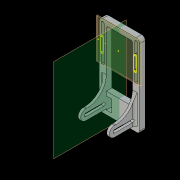
# Autodesk Inventor part: VSlider
Saved by Autodesk Inventor 2022 (Build 260153000, 153)
## iProperties
Created: 2021-12-03
Part Number: VSlider
Material: Generic
Document SubType Name: Modeling
Designer: alber
Density: 1 g/cm^3
Appearance: Default
Mass: 67.3416 g
Surface Area: 306.613 cm^2
Volume: 67.3416 cm^3
Author: alber
Autodesk Inventor part; units mm, degrees
ref_plane "YZ Plane" through (0, 0, 0) normal (1, 0, 0) x (0, 1, 0)
ref_plane "XZ Plane" through (0, 0, 0) normal (0, 1, 0) x (-1, 0, 0)
ref_plane "XY Plane" through (0, 0, 0) normal (0, 0, 1) x (1, 0, 0)
ref_plane "Work Plane1" through (0, 0, 0) normal (0, 0, 1) x (1, 0, 0)
sketch "Sketch1" plane through (0, 0, 0) normal (0, 0, 1) x (1, 0, 0)
  arc A0 (29.8457, -17.7) -> (34.8457, -17.7) centre (32.3457, -17.7) ccw projected
  line L0 (34.8457, 8.3) -> (34.8457, -17.7) projected
  line L1 (29.8457, -17.7) -> (29.8457, 8.3) projected
  arc A1 (34.8457, 8.3) -> (29.8457, 8.3) centre (32.3457, 8.3) ccw projected
  arc A2 (-34.8457, -17.7) -> (-29.8457, -17.7) centre (-32.3457, -17.7) ccw projected
  line L2 (-29.8457, 8.3) -> (-29.8457, -17.7) projected
  line L3 (-34.8457, -17.7) -> (-34.8457, 8.3) projected
  arc A3 (-29.8457, 8.3) -> (-34.8457, 8.3) centre (-32.3457, 8.3) ccw projected
  point P0 (0, 0)
ref_plane "Work Plane2" through (0, 0, -2) normal (0, 0, -1) x (-1, 0, 0)
sketch "Sketch2" plane through (0, 0, -2) normal (0, 0, -1) x (-1, 0, 0)
  arc A0 (-24.3457, -33) -> (-22.3457, -35) centre (-22.3457, -33) ccw projected
  line L0 (-24.3457, -33) -> (-24.3457, -31.7) projected
  arc A1 (-24.3457, -31.7) -> (-31.3457, -24.7) centre (-31.3457, -31.7) ccw projected
  line L1 (-31.3457, -24.7) -> (-32.3457, -24.7) projected
  arc A2 (-39.3457, -17.7) -> (-32.3457, -24.7) centre (-32.3457, -17.7) ccw projected
  line L2 (-39.3457, -17.7) -> (-39.3457, 8.3) projected
  arc A3 (-32.3457, 15.3) -> (-39.3457, 8.3) centre (-32.3457, 8.3) ccw projected
  line L3 (-32.3457, 15.3) -> (-31.3457, 15.3) projected
  arc A4 (-31.3457, 15.3) -> (-24.3457, 22.3) centre (-31.3457, 22.3) ccw projected
  line L4 (-24.3457, 22.3) -> (-24.3457, 33) projected
  arc A5 (-22.3457, 35) -> (-24.3457, 33) centre (-22.3457, 33) ccw projected
  line L5 (-22.3457, 35) -> (22.3457, 35) projected
  arc A6 (24.3457, 33) -> (22.3457, 35) centre (22.3457, 33) ccw projected
  line L6 (24.3457, 33) -> (24.3457, 22.3) projected
  arc A7 (24.3457, 22.3) -> (31.3457, 15.3) centre (31.3457, 22.3) ccw projected
  line L7 (31.3457, 15.3) -> (32.3457, 15.3) projected
  arc A8 (39.3457, 8.3) -> (32.3457, 15.3) centre (32.3457, 8.3) ccw projected
  line L8 (39.3457, 8.3) -> (39.3457, -17.7) projected
  arc A9 (32.3457, -24.7) -> (39.3457, -17.7) centre (32.3457, -17.7) ccw projected
  line L9 (32.3457, -24.7) -> (31.3457, -24.7) projected
  arc A10 (31.3457, -24.7) -> (24.3457, -31.7) centre (31.3457, -31.7) ccw projected
  line L10 (24.3457, -31.7) -> (24.3457, -33) projected
  arc A11 (22.3457, -35) -> (24.3457, -33) centre (22.3457, -33) ccw projected
  line L11 (22.3457, -35) -> (-22.3457, -35) projected
  circle A12 centre (0, 0) radius 13 projected
  line L12 (-29.8457, -17.7) -> (-29.8457, 8.3) projected
  arc A13 (-29.8457, 8.3) -> (-34.8457, 8.3) centre (-32.3457, 8.3) ccw projected
  line L13 (-34.8457, 8.3) -> (-34.8457, -17.7) projected
  arc A14 (-34.8457, -17.7) -> (-29.8457, -17.7) centre (-32.3457, -17.7) ccw projected
  circle A15 centre (15.5, 15.5) radius 2.2 projected
  circle A16 centre (15.5, -15.5) radius 2.2 projected
  arc A17 (34.8457, 8.3) -> (29.8457, 8.3) centre (32.3457, 8.3) ccw projected
  line L14 (29.8457, 8.3) -> (29.8457, -17.7) projected
  arc A18 (29.8457, -17.7) -> (34.8457, -17.7) centre (32.3457, -17.7) ccw projected
  line L15 (34.8457, -17.7) -> (34.8457, 8.3) projected
  circle A19 centre (-15.5, -15.5) radius 2.2 projected
  circle A20 centre (-15.5, 15.5) radius 2.2 projected
  line L16 (-25.5, 15.5) -> (-25.5, -15.5) projected
  line L17 (-39.3457, -122.4215) -> (-29.8457, -122.4215)
  line L18 (-25.5, -104.7632) -> (-25.5, 30.869)
  line L19 (-34.8457, 37.4807) -> (-34.9228, 37.4807)
  line L20 (-39.3457, 30.869) -> (-39.3457, -104.7632)
  arc A21 (-29.9228, 30.2322) -> (-34.9228, 30.2322) centre (-32.4228, 30.2322) ccw
  arc A22 (-34.9228, -104.7632) -> (-29.9228, -104.7632) centre (-32.4228, -104.7632) ccw
  line L21 (-34.9228, -104.7632) -> (-34.9228, 30.2322)
  line L22 (-29.9228, 30.2322) -> (-29.9228, -104.7632)
  arc A23 (-39.3457, -104.7632) -> (-25.5, -104.7632) centre (-32.4228, -104.7632) ccw
  line L23 (-25.2868, -104.7632) -> (-29.9228, -104.7632)
  line L24 (-34.9228, -104.7632) -> (-39.3457, -104.7632)
  arc A24 (-25.5, 30.2322) -> (-39.3457, 30.2322) centre (-32.4228, 30.5506) ccw
  line L25 (-25.5, 30.2322) -> (-29.9228, 30.2322)
  line L26 (-34.9228, 30.2322) -> (-39.3457, 30.2322)
  point P0 (0, 0)
  point P1 (-39.3457, -17.7)
  point P2 (-29.9228, 8.9164)
  point P3 (-29.9228, -18.3164)
  dimension "d0" = 5
  dimension "d1" = 5
  constraints: 20 end point, 10 point on circle, 7 point on line, 4 centre point, 3 horizontal, 3 perpendicular, 2 tangent, 1 concentric, 1 parallel
  measures "d0" diameter of A21
  measures "d1" diameter of A22
extrude "Extrusion1" add sketch "Sketch2" along normal blind 7 contours L18 L23 L22 A1 | A1 L22 A14 L12 A13 A4 L18 L16 | A23 L24 A22 L23 | L20 A2 L21 L24 | L2 A3 L21 A2 | A4 L22 L25 L18 | L20 L26 L21 A3 | L25 A21 L26 L20 A24 L18
mirror "Mirror1" about plane through (0, 0, 0) normal (1, 0, 0) of "Extrusion1"
sketch "Sketch3" plane through (0, 0, -2) normal (0, 0, 1) x (1, 0, 0)
  arc A0 (39.3457, 30.869) -> (25.5, 30.869) centre (32.4228, 30.5506) ccw projected
  arc A1 (-25.5, 30.869) -> (-39.3457, 30.869) centre (-32.4228, 30.5506) ccw projected
  arc A2 (39.3457, 30.869) -> (25.5, 30.869) centre (32.4228, 30.5506) ccw projected
  line L0 (32.4228, 37.4807) -> (-32.4228, 37.4807)
  line L1 (32.4228, 32.4807) -> (-32.4228, 32.4807)
  point P0 (0, 0)
  point P1 (-25.7669, 32.4807)
  point P2 (25.7669, 32.4807)
  dimension "d4" = 5
  constraints: 4 end point, 3 point on circle, 1 parallel
  measures "d4" distance between parallel lines of L0 L1
extrude "Extrusion2" add sketch "Sketch3" against normal blind 7
fillet "Fillet1" radius 5 2 edges at (25.7669, 32.4807, -5.5) (-25.7669, 32.4807, -5.5)
sketch "Sketch4" plane through (-39.3457, -104.7632, -2) normal (-1, 0, 0) x (0, 0, 1)
  point P0 (2, 104.7632)
sketch "Sketch5" plane through (25.5, -104.7632, -9) normal (-1, 0, 0) x (0, 0, 1)
  line L0 (7, -6.9228) -> (7, 0) projected
  line L1 (7, -6.9228) -> (47, -6.9228)
  line L2 (47, 13.0772) -> (7, 13.0772)
  line L3 (7, 13.0772) -> (7, -6.9228)
  circle A0 centre (47, 3.0772) radius 3
  circle A1 centre (12, 3.0774) radius 3
  line L4 (46.9982, 6.0772) -> (12, 6.0774)
  line L5 (0, 0) -> (0, 135.6321) projected
  line L6 (7, -7.5344) -> (0, -7.5344)
  line L7 (0, -7.5344) -> (0, 13.0772)
  line L8 (0, 13.0772) -> (7, 13.0772)
  line L9 (7, 13.0772) -> (7, -7.5344)
  arc A2 (47, -6.9228) -> (47, 13.0772) centre (47, 3.0772) ccw
  line L10 (46.9009, 0.0788) -> (12.0001, 0.0774)
  point P0 (9, 104.7632)
  point P1 (9.4182, 1.5496)
  dimension "d10" = 6
  dimension "d11" = 6
  dimension "d47" = 40
  dimension "d49" = 10
  dimension "d50" = 5
  constraints: 18 end point, 7 point on circle, 4 tangent, 3 centre point, 3 parallel, 2 horizontal, 1 concentric, 1 perpendicular, 1 point on line
  measures "d10" diameter of A0
  measures "d11" diameter of A1
  measures "d47" distance of L0.start L1.end
  measures "d49" radius of A2
  measures "d50" distance from line of L0 A1.centre
extrude "Extrusion3" add sketch "Sketch5" against normal blind 5
sketch "Sketch6" plane through (0, 0, -9) normal (0, 0, -1) x (-1, 0, 0)
  line L0 (-25.5, -112.2975) -> (-30.5, -112.2975) projected
  line L1 (-25.5, 30.869) -> (-25.5, -112.2975) projected
  line L2 (-39.3457, 30.869) -> (-39.3457, -104.7632) projected
  line L3 (-25.5, -91.686) -> (-30.5, -91.686) projected
  line L4 (-25.5, -91.686) -> (-39.3457, -91.686)
  line L5 (-39.3457, -91.686) -> (-39.3457, -112.2975)
  line L6 (-39.3457, -112.2975) -> (-25.5, -112.2975)
  line L7 (-25.5, -112.2975) -> (-25.5, -91.686)
  point P0 (0, 0)
  constraints: 8 end point, 2 parallel, 1 horizontal, 1 perpendicular
extrude "Extrusion4" add sketch "Sketch6" against normal up to surface (7 mm away)
sketch "Sketch7" plane through (25.5, -112.2975, -9) normal (0, -1, 0) x (1, 0, 0)
  line L0 (0, 0) -> (0, 7) projected
  line L1 (0, 0) -> (13.8457, 0) projected
  line L2 (13.8457, 0) -> (13.8457, 7) projected
  line L3 (0, 7) -> (13.8457, 7) projected
  point P0 (-25.5, 9)
extrude "Extrusion5" cut sketch "Sketch7" against normal up to surface (0.6115 mm away)
fillet "Fillet2" radius 4 1 edges at (30.5, -101.686, -2)
ref_plane "Work Plane3" through (0, -104.7632, -2) normal (-1, 0, 0) x (0, 0, 1)
mirror "Mirror2" about plane through (0, -104.7632, -2) normal (-1, 0, 0) of "Extrusion3", "Fillet2", "Extrusion5", "Extrusion4"
sketch "Sketch8" plane through (-25.5, 30.869, -2) normal (1, 0, 0) x (0, 0, -1)
  point P0 (-2, -30.869)
sketch "Sketch9" plane through (-25.5, 30.869, -2) normal (1, 0, 0) x (0, 0, -1)
  line L0 (7, 0) -> (7, -142.555) projected
  line L1 (0, -122.555) -> (0, 0) projected
  line L2 (7, -142.555) -> (0, -142.555)
  line L3 (0, -142.555) -> (0, -122.555)
  line L4 (0, -122.555) -> (7, -122.555)
  line L5 (7, -122.555) -> (7, -142.555)
  point P0 (-2, -30.869)
  constraints: 8 end point, 2 parallel, 1 horizontal, 1 perpendicular
extrude "Extrusion6" add sketch "Sketch9" along normal up to surface (51 mm away)
sketch "Sketch10" plane through (-34.9228, 30.2322, -2) normal (1, 0, 0) x (0, 0, -1)
  line L0 (0, -121.9182) -> (7, -121.9182) projected
  line L1 (7, -121.9182) -> (7, 0) projected
  line L2 (0, -121.9182) -> (7, -121.9182)
  line L3 (7, -121.9182) -> (7, -117.3409)
  line L4 (7, -117.3409) -> (0, -117.3409)
  line L5 (0, -117.3409) -> (0, -121.9182)
  point P0 (-2, -30.2322)
  constraints: 8 end point, 2 parallel, 1 horizontal, 1 perpendicular, 1 point on line
extrude "Extrusion7" add sketch "Sketch10" along normal up to surface (5 mm away)
mirror "Mirror3" about plane through (0, -104.7632, -2) normal (-1, 0, 0) of "Extrusion7"
sketch "Sketch11" plane through (-39.3457, -111.686, -9) normal (0, -1, 0) x (1, 0, 0)
  line L0 (0, 0) -> (0, 7) projected
  line L1 (78.6913, 0) -> (64.8457, 0) projected
  line L2 (0, 7) -> (78.6913, 7)
  line L3 (78.6913, 7) -> (78.6913, 0)
  line L4 (78.6913, 0) -> (0, 0)
  line L5 (0, 0) -> (0, 7)
  point P0 (39.3457, 9)
  constraints: 8 end point, 2 parallel, 1 horizontal, 1 perpendicular
extrude "Extrusion8" add sketch "Sketch11" along normal blind 10
move faces "Move1" translate (0, 10, 0) faces at (-8.5, -91.686, -6.6667)
sketch "Sketch12" plane through (0, 0, -2) normal (0, 0, 1) x (1, 0, 0)
  line L0 (-25.5, -91.686) -> (-34.5, -91.686) projected
  line L1 (-15.5, -113.686) -> (-25.5, -113.686)
  line L2 (-25.5, -113.686) -> (-15.5, -113.686)
  line L3 (-15.5, -113.686) -> (-15.5, -89.686)
  line L4 (-15.5, -89.686) -> (-25.5, -89.686)
  line L5 (-25.5, -89.686) -> (-25.5, -113.686)
  line L6 (-25.5, -81.686) -> (25.5, -81.686) projected
  line L7 (0, -81.686) -> (0, -121.686)
  line L8 (39.3457, -121.686) -> (-39.3457, -121.686) projected
  line L9 (15.5, -113.686) -> (25.5, -113.686)
  line L10 (15.5, -113.686) -> (15.5, -89.686)
  line L11 (15.5, -89.686) -> (25.5, -89.686)
  line L12 (25.5, -89.686) -> (25.5, -113.686)
  point P0 (0, 0)
  dimension "d30" = 10
  dimension "d32" = 10
  dimension "d33" = 24
  constraints: 20 end point, 5 symmetric about line, 2 midpoint, 2 parallel, 1 horizontal, 1 perpendicular
  measures "d30" distance of L1.start L1.end
  measures "d32" distance of L4.end L3.end
  measures "d33" distance of L3.end L2.end
extrude "Extrusion9" cut sketch "Sketch12" against normal blind 13.8125
move faces "Move2" translate (0, 12.7, 0) faces at (33.2562, -87.1087, -6.6667) (-33.2562, -87.1087, -6.6667)
move faces "Move3" translate (0, -3.175, 0) faces at (-18.8333, -89.686, -4.3333) (22.1667, -89.686, -6.6667)
fillet "Fillet6" radius 37.6375 2 edges at (-30, -91.686, -2) (30, -91.686, -2)
move faces "Move4" translate (0, 3, 0) faces at (-18.8333, -92.861, -4.3333) (22.1667, -92.861, -4.3333)
fillet "Fillet7" radius 5 2 edges at (-39.3457, -121.686, -5.5) (39.3457, -121.686, -5.5)
sketch "Sketch13" plane through (-21.823, 32.4807, -2) normal (0, -1, 0) x (1, 0, 0)
  line L0 (0, -7) -> (-3.677, -7) projected
  line L1 (0, -7) -> (0, 0) projected
  line L2 (0, 0) -> (-3.677, 0) projected
  line L3 (-3.677, 0) -> (-3.677, -7) projected
  line L4 (0, -7) -> (0, 0) projected
  line L5 (43.6461, -7) -> (0, -7) projected
  line L6 (43.6461, 0) -> (43.6461, -7) projected
  line L7 (0, 0) -> (43.6461, 0) projected
  line L8 (43.6461, 0) -> (47.323, 0) projected
  line L9 (43.6461, 0) -> (43.6461, -7) projected
  line L10 (43.6461, -7) -> (47.323, -7) projected
  line L11 (47.323, 0) -> (47.323, -7) projected
  point P0 (21.823, 2)
extrude "Extrusion10" add sketch "Sketch13" along normal blind 4
fillet "Fillet8" radius 3 2 edges at (-25.5, 28.4807, -5.5) (25.5, 28.4807, -5.5)
sketch "Sketch14" plane through (0, 0, -9) normal (0, 0, -1) x (-1, 0, 0)
  line L0 (-34.9228, -74.4087) -> (-34.9228, 30.2322) projected
  arc A0 (-29.9228, 30.2322) -> (-34.9228, 30.2322) centre (-32.4228, 30.2322) ccw projected
  line L1 (-29.9228, 30.2322) -> (-29.9228, 8.9164) projected
  arc A1 (-29.8457, 8.3) -> (-29.9228, 8.9164) centre (-32.3457, 8.3) ccw projected
  line L2 (-29.8457, 8.3) -> (-29.8457, -17.7) projected
  arc A2 (-29.9228, -18.3164) -> (-29.8457, -17.7) centre (-32.3457, -17.7) ccw projected
  line L3 (-29.9228, -18.3164) -> (-29.9228, -74.4087) projected
  line L4 (-34.9228, -74.4087) -> (-29.9228, -74.4087) projected
  line L5 (29.9228, -18.3164) -> (29.9228, -74.4087) projected
  arc A3 (29.8457, -17.7) -> (29.9228, -18.3164) centre (32.3457, -17.7) ccw projected
  line L6 (29.8457, 8.3) -> (29.8457, -17.7) projected
  arc A4 (29.9228, 8.9164) -> (29.8457, 8.3) centre (32.3457, 8.3) ccw projected
  line L7 (29.9228, 30.2322) -> (29.9228, 8.9164) projected
  arc A5 (34.9228, 30.2322) -> (29.9228, 30.2322) centre (32.4228, 30.2322) ccw projected
  line L8 (34.9228, -74.4087) -> (34.9228, 30.2322) projected
  line L9 (34.9228, -74.4087) -> (29.9228, -74.4087) projected
  line L10 (25.5, -81.686) -> (25.5, 25.4807) projected
  line L11 (25.5, -81.686) -> (-25.5, -81.686) projected
  arc A6 (-22.5, 28.4807) -> (-25.5, 25.4807) centre (-22.5, 25.4807) ccw projected
  line L12 (22.5, 28.4807) -> (-22.5, 28.4807) projected
  arc A7 (25.5, 25.4807) -> (22.5, 28.4807) centre (22.5, 25.4807) ccw projected
  line L13 (25.5, -113.686) -> (15.5, -113.686) projected
  line L14 (15.5, -113.686) -> (15.5, -89.861) projected
  line L15 (15.5, -89.861) -> (25.5, -89.861) projected
  line L16 (25.5, -89.861) -> (25.5, -113.686) projected
  line L17 (-25.5, -89.861) -> (-15.5, -89.861) projected
  line L18 (-15.5, -89.861) -> (-15.5, -113.686) projected
  line L19 (-15.5, -113.686) -> (-25.5, -113.686) projected
  line L20 (-25.5, -113.686) -> (-25.5, -89.861) projected
  arc A8 (-39.3457, -116.686) -> (-34.3457, -121.686) centre (-34.3457, -116.686) ccw projected
  line L21 (34.3457, -121.686) -> (-34.3457, -121.686) projected
  arc A9 (34.3457, -121.686) -> (39.3457, -116.686) centre (34.3457, -116.686) ccw projected
  line L22 (39.3457, 30.869) -> (39.3457, -116.686) projected
  arc A10 (39.3457, 30.869) -> (32.4228, 37.4807) centre (32.4228, 30.5506) ccw projected
  line L23 (32.4228, 37.4807) -> (-32.4228, 37.4807) projected
  arc A11 (-32.4228, 37.4807) -> (-39.3457, 30.869) centre (-32.4228, 30.5506) ccw projected
  line L24 (-39.3457, 30.869) -> (-39.3457, -116.686) projected
  line L25 (-25.5, -81.686) -> (-25.5, 25.4807) projected
  point P0 (0, 0)
extrude "Extrusion11" add sketch "Sketch14" along normal blind 4
move faces "Move5" translate (0, 34.925, 0) faces at (32.6186, -74.4087, -9.3333) (-32.6186, -74.4087, -9.3333)
body "Solid1"
